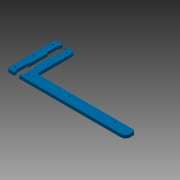
# Autodesk Inventor part: zCar_b
Saved by Autodesk Inventor 2013 (Build 170138000, 138)
## iProperties
Created: 2015-01-14
Part Number: zCar_b
Material: Generic
Document SubType Name: Modeling
Designer: dzban
Density: 1 g/cm^3
Author: dzban
Autodesk Inventor part; units mm, degrees
ref_plane "YZ Plane" through (0, 0, 0) normal (1, 0, 0) x (0, 1, 0)
ref_plane "XZ Plane" through (0, 0, 0) normal (0, 1, 0) x (-1, 0, 0)
ref_plane "XY Plane" through (0, 0, 0) normal (0, 0, 1) x (1, 0, 0)
sketch "Sketch1" plane through (0, 0, 0) normal (0, 0, 1) x (1, 0, 0)
  arc A0 (210.2836, -26.2233) -> (219.2836, -17.2233) centre (210.2836, -17.2233) ccw
  line L0 (219.2836, -17.2233) -> (219.2836, -11.2233)
  arc A1 (219.2836, -11.2233) -> (214.2836, -6.2233) centre (214.2836, -11.2233) ccw
  line L1 (214.2836, -6.2233) -> (29.2836, -6.2233)
  arc A2 (24.2836, -1.2233) -> (29.2836, -6.2233) centre (29.2836, -1.2233) ccw
  line L2 (24.2836, -1.2233) -> (24.2836, 63.7767)
  arc A3 (24.2836, 63.7767) -> (19.2836, 68.7767) centre (19.2836, 63.7767) ccw
  line L3 (19.2836, 68.7767) -> (9.7836, 68.7767)
  line L4 (9.7836, 68.7767) -> (9.7836, 63.7767)
  line L5 (9.7836, 63.7767) -> (12.2836, 63.7767)
  line L6 (12.2836, 63.7767) -> (12.2836, 39.7767)
  line L7 (12.2836, 39.7767) -> (9.7836, 39.7767)
  line L8 (9.7836, 39.7767) -> (9.7836, 2.7767)
  line L9 (9.7836, 2.7767) -> (12.2836, 2.7767)
  line L10 (12.2836, 2.7767) -> (12.2836, -21.2233)
  line L11 (12.2836, -21.2233) -> (9.7836, -21.2233)
  line L12 (9.7836, -21.2233) -> (9.7836, -26.2233)
  line L13 (9.7836, -26.2233) -> (210.2836, -26.2233)
  circle A4 centre (18.5836, 58.7767) radius 1.5
  circle A5 centre (184.4836, -12.4233) radius 1.5
  circle A6 centre (94.8836, -12.4233) radius 1.5
  circle A7 centre (18.5836, -16.2233) radius 1.5
  circle A8 centre (18.5836, 21.2767) radius 1.5
  arc A9 (-14.7164, -21.2233) -> (-9.7164, -26.2233) centre (-9.7164, -21.2233) ccw
  line L14 (-9.7164, -26.2233) -> (-0.2164, -26.2233)
  line L15 (-0.2164, -26.2233) -> (-0.2164, -21.2233)
  line L16 (-0.2164, -21.2233) -> (-2.7164, -21.2233)
  line L17 (-2.7164, -21.2233) -> (-2.7164, 2.7767)
  line L18 (-2.7164, 2.7767) -> (-0.2164, 2.7767)
  line L19 (-0.2164, 2.7767) -> (-0.2164, 39.7767)
  line L20 (-0.2164, 39.7767) -> (-2.7164, 39.7767)
  line L21 (-2.7164, 39.7767) -> (-2.7164, 63.7767)
  line L22 (-2.7164, 63.7767) -> (-0.2164, 63.7767)
  line L23 (-0.2164, 63.7767) -> (-0.2164, 68.7767)
  line L24 (-0.2164, 68.7767) -> (-15.7164, 68.7767)
  line L25 (-15.7164, 68.7767) -> (-15.7164, 65.7767)
  line L26 (-15.7164, 65.7767) -> (-14.7164, 65.7767)
  line L27 (-14.7164, 65.7767) -> (-14.7164, -21.2233)
  circle A10 centre (-9.0164, 21.2767) radius 1.5
  circle A11 centre (-9.0164, -16.2233) radius 1.5
  circle A12 centre (-9.0164, 58.7767) radius 1.5
  point P0 (0, 0)
  point P1 (0, 0)
  constraints: 56 end point, 13 centre point, 10 point on circle
extrude "Extrusion1" add sketch "Sketch1" along normal blind 6
body "Solid1"
